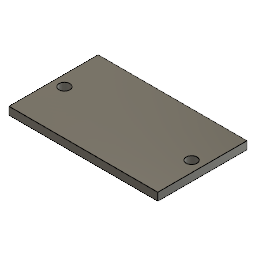
Base v63 (Autodesk Fusion 360 archive; units mm, degrees)
design "Global_I2C_Multiplexer"
Autodesk Fusion 360 part; units mm, degrees
sketch "Sketch1" plane through (0, 0, 0) normal (0, 1, 0) x (1, 0, 0)
  line L0 (-15, -9) -> (15, -9)
  line L1 (15, -9) -> (15, 9)
  line L2 (15, 9) -> (-15, 9)
  line L3 (-15, 9) -> (-15, -9)
  line L4 (-15, -9) -> (15, 9) construction
  line L5 (15, -9) -> (-15, 9) construction
  circle A0 centre (12.8, 0) radius 1.1
  circle A1 centre (-12.8, 0) radius 1.1
  dimension "d1" = 30
  dimension "d2" = 18
  dimension "d3" = 2.2
  dimension "d4" = 2.2
  dimension "d5" = 2.2
  dimension "d6" = 2.2
  constraint perpendicular L0 L1
  constraint parallel L0 L2
  constraint parallel L1 L3
  constraint horizontal L0
  constraint coincident L4 origin
  constraint coincident L5 origin
  measures "d1" distance of L1.end L2.end
  measures "d2" distance of L0.start L2.end
  measures "d3" diameter of A0
  measures "d4" diameter of A1
  measures "d5" distance of L1 A0.centre
  measures "d6" distance of L3 A1.centre
extrude "Extrude1" add sketch "Sketch1" along normal blind 1.6
